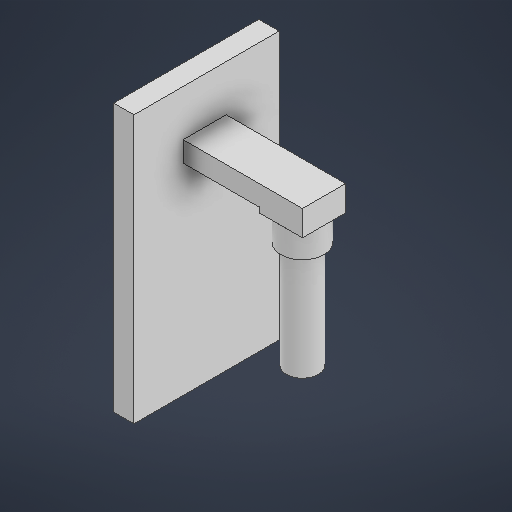
# Autodesk Inventor part: servo_sandboxv2
Saved by Autodesk Inventor 2026.1 (Build 301233020, 233B)
## iProperties
Created: 2026-02-13
Part Number: servo_sandboxv2
Material: Generic
Document SubType Name: Modeling
Designer: Dylan
Density: 1 g/cm^3
Appearance: Default
Author: Dylan
Autodesk Inventor part; units mm, degrees
ref_plane "YZ Plane" through (0, 0, 0) normal (1, 0, 0) x (0, 1, 0)
ref_plane "XZ Plane" through (0, 0, 0) normal (0, 1, 0) x (-1, 0, 0)
ref_plane "XY Plane" through (0, 0, 0) normal (0, 0, 1) x (1, 0, 0)
sketch "Sketch1" plane through (0, 0, 0) normal (0, 1, 0) x (-1, 0, 0)
  circle A0 centre (0, 0) radius 3.135
  dimension "d0" = 6.27
  constraints: 1 centre point, 1 coincident
  measures "d0" diameter of A0
extrude "Extrusion1" add sketch "Sketch1" along normal blind 25
sketch "Sketch3" plane through (0, 25, 0) normal (0, 1, 0) x (1, 0, 0)
  circle A0 centre (0, 0) radius 4.25
  dimension "d3" = 8.5
  constraints: 1 centre point, 1 coincident
  measures "d3" diameter of A0
extrude "Extrusion2" add sketch "Sketch3" against normal blind 4
sketch "Sketch4" plane through (0, 25, 0) normal (0, 1, 0) x (1, 0, 0)
  circle A0 centre (0, 0) radius 3.15
  dimension "d6" = 6.3
  constraints: 1 centre point, 1 coincident
  measures "d6" diameter of A0
extrude "Extrusion3" cut sketch "Sketch4" against normal blind 4.2
sketch "Sketch5" plane through (0, 20.8, 0) normal (0, 1, 0) x (1, 0, 0)
  circle A0 centre (0, 0) radius 3.135
  dimension "d9" = 6.27
  constraints: 1 centre point, 1 coincident
  measures "d9" diameter of A0
extrude "Extrusion4" add sketch "Sketch5" along normal blind 3.5
chamfer "Chamfer1" distance 1.25 angle 45 1 edges at (-3.135, 24.3, 0)
sketch "Sketch6" plane through (0, 25, 0) normal (0, 1, 0) x (1, 0, 0)
  circle A0 centre (0, 0) radius 4.25
  constraints: 1 centre point, 1 coincident
extrude "Extrusion5" add sketch "Sketch6" along normal blind 1
sketch "Sketch7" plane through (0, 26, 0) normal (0, 1, 0) x (1, 0, 0)
  line L0 (4.25, 4.25) -> (-4.25, 4.25)
  line L1 (-4.25, 4.25) -> (-4.25, -4.25)
  line L2 (-4.25, -4.25) -> (4.25, -4.25)
  line L3 (4.25, -4.25) -> (4.25, 4.25)
  point P0 (0, 0)
  constraints: 8 end point, 2 parallel, 1 horizontal, 1 perpendicular
extrude "Extrusion6" add sketch "Sketch7" along normal blind 5
sketch "Sketch8" plane through (-4.25, 26, -4.25) normal (-1, 0, 0) x (0, 0, 1)
  line L0 (8.5, 0) -> (8.5, 5) projected
  line L1 (0, 0) -> (0, 5) projected
  line L2 (8.5, 5) -> (0, 5)
  line L3 (0, 5) -> (0, 1)
  line L4 (0, 1) -> (8.5, 1)
  line L5 (8.5, 1) -> (8.5, 5)
  point P0 (4.25, -26)
  point P1 (8.5, 1)
  dimension "d19" = 4
  constraints: 8 end point, 2 parallel, 1 horizontal, 1 perpendicular, 1 point on line
  measures "d19" distance of L3.end L2.end
extrude "Extrusion7" add sketch "Sketch8" along normal blind 15
sketch "Sketch9" plane through (-19.25, 26, -4.25) normal (-1, 0, 0) x (0, 0, 1)
  line L0 (-10.401, 14.0857) -> (18.1917, 14.0857)
  line L1 (18.1917, 14.0857) -> (18.1917, -38.6412)
  line L2 (18.1917, -38.6412) -> (-10.401, -38.6412)
  line L3 (-10.401, -38.6412) -> (-10.401, 14.0857)
  point P0 (4.25, -26)
  constraints: 8 end point, 2 parallel, 1 horizontal, 1 perpendicular
extrude "Extrusion8" add sketch "Sketch9" along normal blind 4
body "Solid1"
